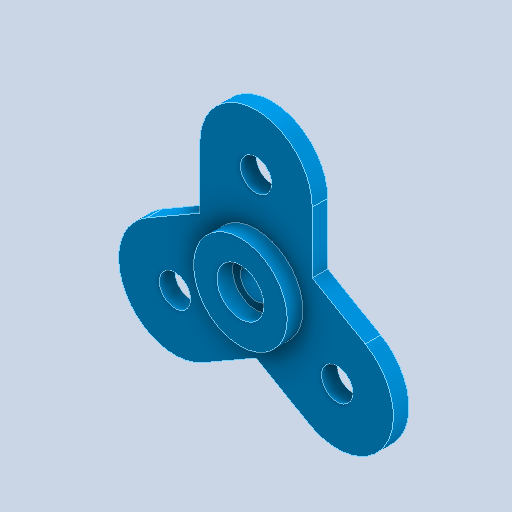
# Autodesk Inventor part: joint3_carrier
Saved by Autodesk Inventor 2025.3 (Build 293356030, 356C)
## iProperties
Created: 2025-09-07
Part Number: joint3_carrier
Material: PLA+ filament
Document SubType Name: Modeling
Designer: MSI
Density: 1.23 g/cm^3
Appearance: 일반
Mass: 27.1929 g
Surface Area: 105.546 cm^2
Volume: 22.1081 cm^3
Author: MSI
Autodesk Inventor part; units mm, degrees
ref_plane "YZ Plane" through (0, 0, 0) normal (1, 0, 0) x (0, 1, 0)
ref_plane "XZ Plane" through (0, 0, 0) normal (0, 1, 0) x (-1, 0, 0)
ref_plane "XY Plane" through (0, 0, 0) normal (0, 0, 1) x (1, 0, 0)
sketch "스케치1" plane through (0, 0, 0) normal (0, 0, 1) x (1, 0, 0)
  line L0 (0, 0) -> (0, 30) construction
  line L1 (-18, 0) -> (-18, 30)
  line L2 (18, 30) -> (18, 0)
  arc A0 (-18, 0) -> (18, 0) centre (0, 0) ccw
  arc A1 (18, 30) -> (-18, 30) centre (0, 30) ccw
  point P0 (0, 15)
  dimension "d0" = 30
  dimension "d1" = 18
  constraints: 8 end point, 4 point on circle, 4 tangent, 2 centre point, 1 midpoint, 1 parallel, 1 vertical
  measures "d0" distance of L2.start L2.end
  measures "d1" radius of A0
extrude "돌출1" add sketch "스케치1" along normal blind 5
pattern_circular "원형 패턴1" count 3 over 360 about axis through (0, 0, -10) along (0, 0, 1) of "돌출1"
sketch "스케치2" plane through (0, 0, 5) normal (0, 0, 1) x (1, 0, 0)
  arc A0 (16.9808, -30.5885) -> (34.9808, 0.5885) centre (25.9808, -15) ccw projected
  arc A1 (18, 30) -> (-18, 30) centre (0, 30) ccw projected
  arc A2 (-34.9808, 0.5885) -> (-16.9808, -30.5885) centre (-25.9808, -15) ccw projected
  point P0 (0, 0)
  constraints: 3 coincident
hole "구멍1" at (25.9808, -15, 5) at (0, 30, 5) at (-25.9808, -15, 5) direction (0, 0, -1) diameter 10 end through all
sketch "스케치3" plane through (0, 0, 5) normal (0, 0, 1) x (1, 0, 0)
  circle A0 centre (0, 0) radius 15
  dimension "d14" = 30
  constraints: 1 centre point, 1 coincident
  measures "d14" diameter of A0
extrude "돌출2" add sketch "스케치3" along normal blind 5
sketch "스케치4" plane through (0, 0, 10) normal (0, 0, 1) x (1, 0, 0)
  circle A0 centre (0, 0) radius 15 projected
  constraints: 1 coincident
hole "구멍2" at (0, 0, 10) direction (0, 0, -1) diameter 10 end through all counterbore diameter 15 counterbore depth 5
